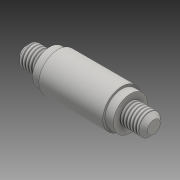
# Autodesk Inventor part: čep háku
Saved by Autodesk Inventor 2016 (Build 200138000, 138)
## iProperties
Created: 2018-11-24
Part Number: čep háku
Material: Generic
Document SubType Name: Modeling
Designer: Radek
Density: 1 g/cm^3
Appearance: Default
Author: Radek
Autodesk Inventor part; units mm, degrees
ref_plane "YZ Plane" through (0, 0, 0) normal (1, 0, 0) x (0, 1, 0)
ref_plane "XZ Plane" through (0, 0, 0) normal (0, 1, 0) x (-1, 0, 0)
ref_plane "XY Plane" through (0, 0, 0) normal (0, 0, 1) x (1, 0, 0)
sketch "Náčrt1" plane through (0, 0, 0) normal (0, 0, 1) x (1, 0, 0)
  line L0 (0, 0) -> (0, 5)
  line L1 (0, 5) -> (11, 5)
  line L2 (11, 5) -> (11, 8)
  line L3 (11, 8) -> (15, 8)
  line L4 (15, 8) -> (15, 9)
  line L5 (15, 9) -> (45, 9)
  line L6 (45, 9) -> (45, 8)
  line L7 (45, 8) -> (49, 8)
  line L8 (49, 8) -> (49, 5)
  line L9 (49, 5) -> (60, 5)
  line L10 (60, 5) -> (60, 0)
  line L11 (60, 0) -> (0, 0)
  dimension "d0" = 11
  dimension "d1" = 15
  dimension "d2" = 10
  dimension "d3" = 16
  dimension "d4" = 18
  dimension "d5" = 45
  constraints: 24 end point, 7 perpendicular, 4 point on line, 2 collinear, 2 vertical, 1 parallel
  measures "d0" distance of L0.end L1.end
  measures "d1" distance between parallel lines of L0 L4
  measures "d2" diameter of L1 L11
  measures "d3" diameter of L3 L11
  measures "d4" diameter of L5 L11
  measures "d5" distance between parallel lines of L0 L6
revolve "Rotace1" add sketch "Náčrt1" angle 360 about axis through (60, 0, 0) along (-1, 0, 0)
chamfer "Zkosení1" distance 2 angle 45 2 edges at (0, -5, 0) (60, -5, 0)
thread "Závit1" size "M10x1.5" class "6g" standard "ANSI Metric M Profile" full length
thread "Závit2" size "M10x1.5" class "6g" standard "ANSI Metric M Profile" full length
